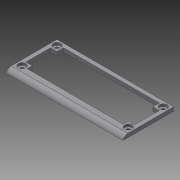
# Autodesk Inventor part: LineTraceCoverFlont
Saved by Autodesk Inventor 2015 (Build 190159000, 159)
## iProperties
Created: 2015-11-15
Part Number: LineTraceCoverFlont
Material: 一般
Document SubType Name: Modeling
Designer: kenta
Density: 1 g/cm^3
Appearance: 既定
Author: kenta
Autodesk Inventor part; units mm, degrees
ref_plane "YZ Plane" through (0, 0, 0) normal (1, 0, 0) x (0, 1, 0)
ref_plane "XZ Plane" through (0, 0, 0) normal (0, 1, 0) x (-1, 0, 0)
ref_plane "XY Plane" through (0, 0, 0) normal (0, 0, 1) x (1, 0, 0)
sketch "スケッチ1" plane through (0, 0, 0) normal (0, 0, 1) x (1, 0, 0)
  line L0 (-45, 3.5) -> (45, 3.5)
  line L1 (45, 3.5) -> (45, -3.5)
  line L2 (45, -3.5) -> (-45, -3.5)
  line L3 (-45, -3.5) -> (-45, 3.5)
  line L4 (-45, 3.5) -> (45, -3.5) construction
  line L5 (45, 3.5) -> (-45, -3.5) construction
  point P0 (0, 0)
  dimension "d0" = 90
  dimension "d1" = 7
  constraints: 12 end point, 2 midpoint, 2 parallel, 1 horizontal, 1 perpendicular
  measures "d0" distance of L1.end L2.end
  measures "d1" distance of L0.end L1.end
extrude "押し出し1" add sketch "スケッチ1" along normal blind 3
sketch "スケッチ2" plane through (0, 0, 3) normal (0, 0, 1) x (1, 0, 0)
  circle A0 centre (-41, -0.4) radius 2.9
  circle A1 centre (41, -0.4) radius 2.9
  line L0 (45, 3.5) -> (-45, 3.5) projected
  line L1 (45, -3.5) -> (45, 3.5) projected
  point P0 (0, 0)
  dimension "d4" = 5.8
  dimension "d5" = 5.8
  dimension "d7" = 3.9
  dimension "d8" = 3.9
  dimension "d9" = 82
  dimension "d10" = 4
  constraints: 2 centre point
  measures "d4" diameter of A1
  measures "d5" diameter of A0
  measures "d7" distance from line of L0 A0.centre
  measures "d8" distance from line of A1.centre L0
  measures "d9" distance of A0.centre A1.centre
  measures "d10" distance from line of A1.centre L1
extrude "押し出し2" cut sketch "スケッチ2" against normal blind 2
sketch "スケッチ3" plane through (0, 0, 0) normal (0, 0, -1) x (-1, 0, 0)
  circle A0 centre (41, -0.4) radius 1.5
  circle A1 centre (-41, -0.4) radius 1.5
  line L0 (45, -3.5) -> (45, 3.5) projected
  line L1 (-45, 3.5) -> (-45, -3.5) projected
  line L2 (45, 3.5) -> (-45, 3.5) projected
  point P0 (0, 0)
  dimension "d13" = 3
  dimension "d14" = 3
  dimension "d15" = 4
  dimension "d16" = 4
  dimension "d17" = 3.9
  dimension "d18" = 3.9
  constraints: 2 centre point
  measures "d13" diameter of A1
  measures "d14" diameter of A0
  measures "d15" distance from line of L0 A0.centre
  measures "d16" distance from line of A1.centre L1
  measures "d17" distance from line of A1.centre L2
  measures "d18" distance from line of A0.centre L2
extrude "押し出し3" cut sketch "スケッチ3" against normal blind 2
sketch "スケッチ4" plane through (-45, -3.5, 0) normal (0, -1, 0) x (1, 0, 0)
  line L0 (0, 0) -> (90, 0)
  line L1 (90, 0) -> (90, 3)
  line L2 (90, 3) -> (0, 3)
  line L3 (0, 3) -> (0, 0)
  point P0 (45, 0)
  constraints: 8 end point, 2 parallel, 1 horizontal, 1 perpendicular
extrude "押し出し4" add sketch "スケッチ4" along normal blind 5
fillet "フィレット1" radius 4 1 edges at (0, -8.5, 3)
sketch "スケッチ6" plane through (0, 0, 0) normal (0, 0, -1) x (-1, 0, 0)
  line L0 (37, -0.5) -> (-37, -0.5)
  line L1 (-37, -0.5) -> (-37, 3.5)
  line L2 (-37, 3.5) -> (37, 3.5)
  line L3 (37, 3.5) -> (37, -0.5)
  line L4 (45, -8.5) -> (45, 3.5) projected
  line L5 (45, 3.5) -> (-45, 3.5) projected
  point P0 (0, 0)
  dimension "d24" = 74
  dimension "d25" = 8
  dimension "d26" = 0
  dimension "d27" = 4
  constraints: 8 end point, 2 parallel, 1 horizontal, 1 perpendicular
  measures "d24" distance of L1.end L2.end
  measures "d25" distance between parallel lines of L4 L3
  measures "d26" distance between parallel lines of L5 L2
  measures "d27" distance of L0.end L1.end
extrude "押し出し5" cut sketch "スケッチ6" against normal blind 10
sketch "スケッチ7" plane through (45, 3.5, 3) normal (0, 1, 0) x (1, 0, 0)
  line L0 (0, 3) -> (-3, 3)
  line L1 (-3, 3) -> (-3, 0)
  line L2 (-3, 0) -> (0, 0)
  line L3 (0, 0) -> (0, 3)
  line L4 (-90, 0) -> (-87, 0)
  line L5 (-87, 0) -> (-87, 3)
  line L6 (-87, 3) -> (-90, 3)
  line L7 (-90, 3) -> (-90, 0)
  point P0 (-45, 3)
  dimension "d30" = 3
  dimension "d31" = 3
  dimension "d32" = 3
  dimension "d33" = 3
  constraints: 16 end point, 4 parallel, 2 horizontal, 2 perpendicular
  measures "d30" distance of L2.end L1.end
  measures "d31" distance of L1.end L0.end
  measures "d32" distance of L6.end L5.end
  measures "d33" distance of L5.end L4.end
extrude "押し出し6" add sketch "スケッチ7" along normal blind 27.1
sketch "スケッチ8" plane through (-42, 3.5, 3) normal (1, 0, 0) x (0, 0, -1)
  line L0 (0, 27.1) -> (3, 27.1)
  line L1 (3, 27.1) -> (3, 24.1)
  line L2 (3, 24.1) -> (0, 24.1)
  line L3 (0, 24.1) -> (0, 27.1)
  point P0 (3, -3.5)
  dimension "d36" = 3
  dimension "d37" = 3
  constraints: 8 end point, 2 parallel, 1 horizontal, 1 perpendicular
  measures "d36" distance of L1.end L2.end
  measures "d37" distance of L0.end L1.end
extrude "押し出し7" add sketch "スケッチ8" along normal blind 86
sketch "スケッチ9" plane through (0, 0, 3) normal (0, 0, 1) x (1, 0, 0)
  line L0 (-45, 30.6) -> (-37, 30.6)
  line L1 (-37, 30.6) -> (-37, 22.6)
  line L2 (-37, 22.6) -> (-45, 22.6)
  line L3 (-45, 22.6) -> (-45, 30.6)
  line L4 (45, 30.6) -> (37, 30.6)
  line L5 (37, 30.6) -> (37, 22.6)
  line L6 (37, 22.6) -> (45, 22.6)
  line L7 (45, 22.6) -> (45, 30.6)
  point P0 (0, 0)
  dimension "d40" = 8
  dimension "d41" = 8
  dimension "d42" = 8
  dimension "d43" = 8
  constraints: 16 end point, 4 parallel, 2 horizontal, 2 perpendicular
  measures "d40" distance of L1.end L2.end
  measures "d41" distance of L0.end L1.end
  measures "d42" distance of L6.end L5.end
  measures "d43" distance of L5.end L4.end
extrude "押し出し8" add sketch "スケッチ9" against normal blind 3
sketch "スケッチ10" plane through (0, 0, 3) normal (0, 0, 1) x (1, 0, 0)
  circle A0 centre (-41, 26.6) radius 1.5
  circle A1 centre (41, 26.6) radius 1.5
  line L0 (-45, 30.6) -> (45, 30.6) projected
  line L1 (-45, -4.627) -> (-45, 30.6) projected
  line L2 (45, 30.6) -> (45, -4.627) projected
  point P0 (0, 0)
  dimension "d46" = 4
  dimension "d47" = 4
  dimension "d50" = 3
  dimension "d51" = 3
  dimension "d52" = 4
  dimension "d53" = 4
  constraints: 2 centre point
  measures "d46" distance from line of A0.centre L0
  measures "d47" distance from line of L1 A0.centre
  measures "d50" diameter of A1
  measures "d51" diameter of A0
  measures "d52" distance from line of A1.centre L0
  measures "d53" distance from line of A1.centre L2
extrude "押し出し9" cut sketch "スケッチ10" against normal blind 3
sketch "スケッチ11" plane through (0, 0, 3) normal (0, 0, 1) x (1, 0, 0)
  circle A0 centre (-41, 26.6) radius 1.5 projected
  circle A1 centre (-41, 26.6) radius 2.9
  circle A2 centre (41, 26.6) radius 2.9
  line L0 (-45, 30.6) -> (45, 30.6) projected
  line L1 (45, 30.6) -> (45, -4.627) projected
  point P0 (0, 0)
  dimension "d56" = 5.8
  dimension "d57" = 5.8
  dimension "d58" = 4
  dimension "d60" = 4
  constraints: 2 centre point, 1 coincident
  measures "d56" diameter of A1
  measures "d57" diameter of A2
  measures "d58" distance from line of A2.centre L0
  measures "d60" distance from line of A2.centre L1
extrude "押し出し10" cut sketch "スケッチ11" against normal blind 2
